Autodesk Inventor part; units mm, degrees
(part 2 of 2)
sketch "スケッチ3" plane through (0, 0, 5) normal (0, 0, 1) x (1, 0, 0)
  circle A0 centre (23.3432, 24.5782) radius 9 projected
  circle A1 centre (33.2427, 14.6787) radius 2.5 projected
  circle A2 centre (13.4437, 14.6787) radius 2.5 projected
  circle A3 centre (33.2427, 34.4777) radius 2.5 projected
  circle A4 centre (13.4437, 34.4777) radius 2.5 projected
  arc A5 (22.1602, 48.3922) -> (21.7942, 49.4809) centre (16.0401, 46.941) ccw projected
  arc A6 (21.7942, 49.4809) -> (20.6745, 51.446) centre (11.8398, 45.1102) ccw projected
  arc A7 (20.6745, 51.446) -> (19.2464, 51.2656) centre (23.3432, 24.5782) ccw projected
  arc A8 (19.2464, 51.2656) -> (18.6505, 49.0838) centre (29.3792, 47.3259) ccw projected
  arc A9 (18.6505, 49.0838) -> (18.5668, 47.9382) centre (24.8555, 48.0547) ccw projected
  arc A10 (18.5668, 47.9382) -> (18.5978, 47.5862) centre (20.8543, 47.962) ccw projected
  line L0 (18.5978, 47.5862) -> (18.7982, 46.6144) projected
  arc A11 (18.7982, 46.6144) -> (16.71, 46.0782) centre (23.3432, 24.5782) ccw projected
  line L1 (16.71, 46.0782) -> (16.4175, 47.0264) projected
  arc A12 (16.4175, 47.0264) -> (16.275, 47.3498) centre (14.259, 46.2687) ccw projected
  arc A13 (16.275, 47.3498) -> (15.6498, 48.3133) centre (10.7081, 44.4223) ccw projected
  arc A14 (15.6498, 48.3133) -> (14.0766, 49.9382) centre (7.0951, 41.6043) ccw projected
  arc A15 (14.0766, 49.9382) -> (12.7382, 49.4083) centre (23.3432, 24.5782) ccw projected
  arc A16 (12.7382, 49.4083) -> (12.7036, 47.1469) centre (23.5324, 48.1123) ccw projected
  arc A17 (12.7036, 47.1469) -> (12.9075, 46.0165) centre (18.9696, 47.6932) ccw projected
  arc A18 (12.9075, 46.0165) -> (13.025, 45.6833) centre (15.1172, 46.6084) ccw projected
  line L2 (13.025, 45.6833) -> (13.4608, 44.7918) projected
  arc A19 (13.4608, 44.7918) -> (11.5716, 43.7532) centre (23.3432, 24.5782) ccw projected
  line L3 (11.5716, 43.7532) -> (11.0524, 44.5988) projected
  arc A20 (11.0524, 44.5988) -> (10.834, 44.8766) centre (9.1502, 43.3281) ccw projected
  arc A21 (10.834, 44.8766) -> (9.9888, 45.6544) centre (6.1701, 40.6566) ccw projected
  arc A22 (9.9888, 45.6544) -> (8.0609, 46.837) centre (3.3713, 37.0287) ccw projected
  arc A23 (8.0609, 46.837) -> (6.8964, 45.9909) centre (23.3432, 24.5782) ccw projected
  arc A24 (6.8964, 45.9909) -> (7.4253, 43.7919) centre (17.6738, 47.42) ccw projected
  arc A25 (7.4253, 43.7919) -> (7.9038, 42.7477) centre (13.3585, 45.8793) ccw projected
  arc A26 (7.9038, 42.7477) -> (8.1005, 42.4542) centre (9.8969, 43.8706) ccw projected
  line L4 (8.1005, 42.4542) -> (8.7444, 41.6991) projected
  arc A27 (8.7444, 41.6991) -> (7.1728, 40.2233) centre (23.3432, 24.5782) ccw projected
  line L5 (7.1728, 40.2233) -> (6.4596, 40.9132) projected
  arc A28 (6.4596, 40.9132) -> (6.179, 41.128) centre (4.9332, 39.2093) ccw projected
  arc A29 (6.179, 41.128) -> (5.167, 41.6712) centre (2.7111, 35.8807) ccw projected
  arc A30 (5.167, 41.6712) -> (3.0055, 42.3371) centre (0.9025, 31.6707) ccw projected
  arc A31 (3.0055, 42.3371) -> (2.088, 41.228) centre (23.3432, 24.5782) ccw projected
  arc A32 (2.088, 41.228) -> (3.1471, 39.2296) centre (12.1714, 45.2925) ccw projected
  arc A33 (3.1471, 39.2296) -> (3.8703, 38.3373) centre (8.3748, 42.727) ccw projected
  arc A34 (3.8703, 38.3373) -> (4.1338, 38.1019) centre (5.5215, 39.9205) ccw projected
  line L6 (4.1338, 38.1019) -> (4.9452, 37.5306) projected
  arc A35 (4.9452, 37.5306) -> (3.7901, 35.7103) centre (23.3432, 24.5782) ccw projected
  line L7 (3.7901, 35.7103) -> (2.9277, 36.2013) projected
  arc A36 (2.9277, 36.2013) -> (2.6025, 36.3395) centre (1.873, 34.1713) ccw projected
  arc A37 (2.6025, 36.3395) -> (1.4872, 36.6139) centre (0.5485, 30.3946) ccw projected
  arc A38 (1.4872, 36.6139) -> (-0.772, 36.7214) centre (-0.1564, 25.8671) ccw projected
  arc A39 (-0.772, 36.7214) -> (-1.3849, 35.4189) centre (23.3432, 24.5782) ccw projected
  arc A40 (-1.3849, 35.4189) -> (0.138, 33.7468) centre (7.3709, 41.8634) ccw projected
  arc A41 (0.138, 33.7468) -> (1.0604, 33.0623) centre (4.3317, 38.4344) ccw projected
  arc A42 (1.0604, 33.0623) -> (1.3741, 32.8998) centre (2.266, 35.0064) ccw projected
  line L8 (1.3741, 32.8998) -> (2.3021, 32.5483) projected
  arc A43 (2.3021, 32.5483) -> (1.6359, 30.4979) centre (23.3432, 24.5782) ccw projected
  line L9 (1.6359, 30.4979) -> (0.6786, 30.759) projected
  arc A44 (0.6786, 30.759) -> (0.3292, 30.812) centre (0.1618, 28.5305) ccw projected
  arc A45 (0.3292, 30.812) -> (-0.8194, 30.8004) centre (-0.1819, 24.543) ccw projected
  arc A46 (-0.8194, 30.8004) -> (-3.0343, 30.3427) centre (0.2614, 19.9825) ccw projected
  arc A47 (-3.0343, 30.3427) -> (-3.304, 28.9287) centre (23.3432, 24.5782) ccw projected
  arc A48 (-3.304, 28.9287) -> (-1.4131, 27.6878) centre (3.5741, 37.3482) ccw projected
  arc A49 (-1.4131, 27.6878) -> (-0.3495, 27.2542) centre (1.4831, 33.2711) ccw projected
  arc A50 (-0.3495, 27.2542) -> (-0.0052, 27.1749) centre (0.3348, 29.4371) ccw projected
  line L10 (-0.0052, 27.1749) -> (0.9811, 27.0652) projected
  arc A51 (0.9811, 27.0652) -> (0.8457, 24.9135) centre (23.3432, 24.5782) ccw projected
  line L11 (0.8457, 24.9135) -> (-0.1465, 24.9283) projected
  arc A52 (-0.1465, 24.9283) -> (-0.4981, 24.8928) centre (-0.0928, 22.6413) ccw projected
  arc A53 (-0.4981, 24.8928) -> (-1.6076, 24.5959) centre (0.5659, 18.6937) ccw projected
  arc A54 (-1.6076, 24.5959) -> (-3.6391, 23.6018) centre (2.1295, 14.3867) ccw projected
  arc A55 (-3.6391, 23.6018) -> (-3.5487, 22.1652) centre (23.3432, 24.5782) ccw projected
  arc A56 (-3.5487, 22.1652) -> (-1.4087, 21.4335) centre (1.0194, 32.0306) ccw projected
  arc A57 (-1.4087, 21.4335) -> (-0.2706, 21.278) centre (0.008, 27.5616) ccw projected
  arc A58 (-0.2706, 21.278) -> (0.0826, 21.2868) centre (-0.1508, 23.5625) ccw projected
  line L12 (0.0826, 21.2868) -> (1.0651, 21.4258) projected
  arc A59 (1.0651, 21.4258) -> (1.4691, 19.3081) centre (23.3432, 24.5782) ccw projected
  line L13 (1.4691, 19.3081) -> (0.5044, 19.0757) projected
  arc A60 (0.5044, 19.0757) -> (0.1727, 18.9538) centre (1.1252, 16.8739) ccw projected
  arc A61 (0.1727, 18.9538) -> (-0.8282, 18.3903) centre (2.745, 13.2141) ccw projected
  arc A62 (-0.8282, 18.3903) -> (-2.5486, 16.9222) centre (5.3305, 9.4312) ccw projected
  arc A63 (-2.5486, 16.9222) -> (-2.1038, 15.5532) centre (23.3432, 24.5782) ccw projected
  arc A64 (-2.1038, 15.5532) -> (0.151, 15.3767) centre (-0.1326, 26.2447) ccw projected
  arc A65 (0.151, 15.3767) -> (1.292, 15.5092) centre (-0.0008, 21.6646) ccw projected
  arc A66 (1.292, 15.5092) -> (1.6319, 15.6055) centre (0.8399, 17.7517) ccw projected
  line L14 (1.6319, 15.6055) -> (2.549, 15.9845) projected
  arc A67 (2.549, 15.9845) -> (3.467, 14.0338) centre (23.3432, 24.5782) ccw projected
  line L15 (3.467, 14.0338) -> (2.5904, 13.5688) projected
  arc A68 (2.5904, 13.5688) -> (2.2994, 13.3682) centre (3.7392, 11.5905) ccw projected
  arc A69 (2.2994, 13.3682) -> (1.4701, 12.5736) centre (6.2182, 8.4485) ccw projected
  arc A70 (1.4701, 12.5736) -> (0.1688, 10.7237) centre (9.6633, 5.4275) ccw projected
  arc A71 (0.1688, 10.7237) -> (0.9401, 9.5083) centre (23.3432, 24.5782) ccw projected
  arc A72 (0.9401, 9.5083) -> (3.168, 9.8981) centre (0.1905, 20.3542) ccw projected
  arc A73 (3.168, 9.8981) -> (4.2401, 10.3102) centre (1.4572, 15.9507) ccw projected
  arc A74 (4.2401, 10.3102) -> (4.5454, 10.488) centre (3.2446, 12.3698) ccw projected
  line L16 (4.5454, 10.488) -> (5.3395, 11.0832) projected
  arc A75 (5.3395, 11.0832) -> (6.7137, 9.4221) centre (23.3432, 24.5782) ccw projected
  line L17 (6.7137, 9.4221) -> (5.9803, 8.7536) projected
  arc A76 (5.9803, 8.7536) -> (5.7483, 8.487) centre (7.585, 7.1232) ccw projected
  arc A77 (5.7483, 8.487) -> (5.1427, 7.5111) centre (10.7675, 4.6965) ccw projected
  arc A78 (5.1427, 7.5111) -> (4.3423, 5.3957) centre (14.8556, 2.6271) ccw projected
  arc A79 (4.3423, 5.3957) -> (5.3917, 4.4104) centre (23.3432, 24.5782) ccw projected
  arc A80 (5.3917, 4.4104) -> (7.4526, 5.342) centre (1.9683, 14.7291) ccw projected
  arc A81 (7.4526, 5.342) -> (8.3886, 6.0077) centre (4.2903, 10.7789) ccw projected
  arc A82 (8.3886, 6.0077) -> (8.6401, 6.2559) centre (6.9121, 7.7551) ccw projected
  line L18 (8.6401, 6.2559) -> (9.2611, 7.0298) projected
  arc A83 (9.2611, 7.0298) -> (11.0053, 5.7626) centre (23.3432, 24.5782) ccw projected
  line L19 (11.0053, 5.7626) -> (10.4612, 4.9328) projected
  arc A84 (10.4612, 4.9328) -> (10.3028, 4.6169) centre (12.4209, 3.7527) ccw projected
  arc A85 (10.3028, 4.6169) -> (9.9589, 3.521) centre (16.107, 2.1936) ccw projected
  arc A86 (9.9589, 3.521) -> (9.7098, 1.2731) centre (20.5813, 1.2059) ccw projected
  arc A87 (9.7098, 1.2731) -> (10.9712, 0.5796) centre (23.3432, 24.5782) ccw projected
  arc A88 (10.9712, 0.5796) -> (12.7357, 1.9945) centre (5.0893, 9.7228) ccw projected
  arc A89 (12.7357, 1.9945) -> (13.4767, 2.872) centre (8.3207, 6.4742) ccw projected
  arc A90 (13.4767, 2.872) -> (13.6586, 3.175) centre (11.6121, 4.1973) ccw projected
  line L20 (13.6586, 3.175) -> (14.0677, 4.0791) projected
  arc A91 (14.0677, 4.0791) -> (16.0722, 3.2854) centre (23.3432, 24.5782) ccw projected
  line L21 (16.0722, 3.2854) -> (15.7515, 2.3464) projected
  arc A92 (15.7515, 2.3464) -> (15.6767, 2.001) centre (17.9432, 1.6907) ccw projected
  arc A93 (15.6767, 2.001) -> (15.6161, 0.854) centre (21.9012, 1.0973) ccw projected
  arc A94 (15.6161, 0.854) -> (15.9339, -1.3853) centre (26.4805, 1.2534) ccw projected
  arc A95 (15.9339, -1.3853) -> (17.3281, -1.7432) centre (23.3432, 24.5782) ccw projected
  arc A96 (17.3281, -1.7432) -> (18.6853, 0.066) centre (9.3571, 5.6499) ccw projected
  arc A97 (18.6853, 0.066) -> (19.1848, 1.1003) centre (13.2949, 3.307) ccw projected
  arc A98 (19.1848, 1.1003) -> (19.2856, 1.439) centre (17.0492, 1.9202) ccw projected
  line L22 (19.2856, 1.439) -> (19.457, 2.4164) projected
  arc A99 (19.457, 2.4164) -> (21.5959, 2.1462) centre (23.3432, 24.5782) ccw projected
  line L23 (21.5959, 2.1462) -> (21.5188, 1.1568) projected
  arc A100 (21.5188, 1.1568) -> (21.5323, 0.8037) centre (23.8047, 1.0668) ccw projected
  arc A101 (21.5323, 0.8037) -> (21.7589, -0.3223) centre (27.7859, 1.4764) ccw projected
  arc A102 (21.7589, -0.3223) -> (22.6235, -2.4122) centre (32.1826, 2.7664) ccw projected
  arc A103 (22.6235, -2.4122) -> (24.0629, -2.4122) centre (23.3432, 24.5782) ccw projected
  arc A104 (24.0629, -2.4122) -> (24.9276, -0.3223) centre (14.5038, 2.7664) ccw projected
  arc A105 (24.9276, -0.3223) -> (25.1542, 0.8037) centre (18.9005, 1.4764) ccw projected
  arc A106 (25.1542, 0.8037) -> (25.1676, 1.1568) centre (22.8817, 1.0668) ccw projected
  line L24 (25.1676, 1.1568) -> (25.0905, 2.1462) projected
  arc A107 (25.0905, 2.1462) -> (27.2294, 2.4164) centre (23.3432, 24.5782) ccw projected
  line L25 (27.2294, 2.4164) -> (27.4008, 1.439) projected
  arc A108 (27.4008, 1.439) -> (27.5016, 1.1003) centre (29.6373, 1.9202) ccw projected
  arc A109 (27.5016, 1.1003) -> (28.0011, 0.066) centre (33.3915, 3.307) ccw projected
  arc A110 (28.0011, 0.066) -> (29.3583, -1.7432) centre (37.3293, 5.6499) ccw projected
  arc A111 (29.3583, -1.7432) -> (30.7526, -1.3853) centre (23.3432, 24.5782) ccw projected
  arc A112 (30.7526, -1.3853) -> (31.0703, 0.854) centre (20.2059, 1.2534) ccw projected
  arc A113 (31.0703, 0.854) -> (31.0098, 2.001) centre (24.7853, 1.0973) ccw projected
  arc A114 (31.0098, 2.001) -> (30.9349, 2.3464) centre (28.7433, 1.6907) ccw projected
  line L26 (30.9349, 2.3464) -> (30.6142, 3.2854) projected
  arc A115 (30.6142, 3.2854) -> (32.6188, 4.0791) centre (23.3432, 24.5782) ccw projected
  line L27 (32.6188, 4.0791) -> (33.0278, 3.175) projected
  arc A116 (33.0278, 3.175) -> (33.2097, 2.872) centre (35.0743, 4.1973) ccw projected
  arc A117 (33.2097, 2.872) -> (33.9507, 1.9945) centre (38.3658, 6.4742) ccw projected
  arc A118 (33.9507, 1.9945) -> (35.7152, 0.5796) centre (41.5972, 9.7228) ccw projected
  arc A119 (35.7152, 0.5796) -> (36.9766, 1.2731) centre (23.3432, 24.5782) ccw projected
  arc A120 (36.9766, 1.2731) -> (36.7275, 3.521) centre (26.1051, 1.2059) ccw projected
  arc A121 (36.7275, 3.521) -> (36.3836, 4.6169) centre (30.5794, 2.1936) ccw projected
  arc A122 (36.3836, 4.6169) -> (36.2252, 4.9328) centre (34.2655, 3.7527) ccw projected
  line L28 (36.2252, 4.9328) -> (35.6811, 5.7626) projected
  arc A123 (35.6811, 5.7626) -> (37.4253, 7.0298) centre (23.3432, 24.5782) ccw projected
  line L29 (37.4253, 7.0298) -> (38.0463, 6.2559) projected
  arc A124 (38.0463, 6.2559) -> (38.2978, 6.0077) centre (39.7743, 7.7551) ccw projected
  arc A125 (38.2978, 6.0077) -> (39.2338, 5.342) centre (42.3961, 10.7789) ccw projected
  arc A126 (39.2338, 5.342) -> (41.2948, 4.4104) centre (44.7181, 14.7291) ccw projected
  arc A127 (41.2948, 4.4104) -> (42.3441, 5.3957) centre (23.3432, 24.5782) ccw projected
  arc A128 (42.3441, 5.3957) -> (41.5437, 7.5111) centre (31.8308, 2.6271) ccw projected
  arc A129 (41.5437, 7.5111) -> (40.9381, 8.487) centre (35.9189, 4.6965) ccw projected
  arc A130 (40.9381, 8.487) -> (40.7062, 8.7536) centre (39.1015, 7.1232) ccw projected
  line L30 (40.7062, 8.7536) -> (39.9727, 9.4221) projected
  arc A131 (39.9727, 9.4221) -> (41.347, 11.0832) centre (23.3432, 24.5782) ccw projected
  line L31 (41.347, 11.0832) -> (42.141, 10.488) projected
  arc A132 (42.141, 10.488) -> (42.4463, 10.3102) centre (43.4418, 12.3698) ccw projected
  arc A133 (42.4463, 10.3102) -> (43.5185, 9.8981) centre (45.2292, 15.9507) ccw projected
  arc A134 (43.5185, 9.8981) -> (45.7463, 9.5083) centre (46.4959, 20.3542) ccw projected
  arc A135 (45.7463, 9.5083) -> (46.5176, 10.7237) centre (23.3432, 24.5782) ccw projected
  arc A136 (46.5176, 10.7237) -> (45.2163, 12.5736) centre (37.0232, 5.4275) ccw projected
  arc A137 (45.2163, 12.5736) -> (44.387, 13.3682) centre (40.4682, 8.4485) ccw projected
  arc A138 (44.387, 13.3682) -> (44.0961, 13.5688) centre (42.9473, 11.5905) ccw projected
  line L32 (44.0961, 13.5688) -> (43.2195, 14.0338) projected
  arc A139 (43.2195, 14.0338) -> (44.1374, 15.9845) centre (23.3432, 24.5782) ccw projected
  line L33 (44.1374, 15.9845) -> (45.0545, 15.6055) projected
  arc A140 (45.0545, 15.6055) -> (45.3945, 15.5092) centre (45.8465, 17.7517) ccw projected
  arc A141 (45.3945, 15.5092) -> (46.5354, 15.3767) centre (46.6872, 21.6646) ccw projected
  arc A142 (46.5354, 15.3767) -> (48.7902, 15.5532) centre (46.819, 26.2447) ccw projected
  arc A143 (48.7902, 15.5532) -> (49.235, 16.9222) centre (23.3432, 24.5782) ccw projected
  arc A144 (49.235, 16.9222) -> (47.5146, 18.3903) centre (41.356, 9.4312) ccw projected
  arc A145 (47.5146, 18.3903) -> (46.5137, 18.9538) centre (43.9415, 13.2141) ccw projected
  arc A146 (46.5137, 18.9538) -> (46.182, 19.0757) centre (45.5613, 16.8739) ccw projected
  line L34 (46.182, 19.0757) -> (45.2173, 19.3081) projected
  arc A147 (45.2173, 19.3081) -> (45.6213, 21.4258) centre (23.3432, 24.5782) ccw projected
  line L35 (45.6213, 21.4258) -> (46.6038, 21.2868) projected
  arc A148 (46.6038, 21.2868) -> (46.9571, 21.278) centre (46.8372, 23.5625) ccw projected
  arc A149 (46.9571, 21.278) -> (48.0951, 21.4335) centre (46.6784, 27.5616) ccw projected
  arc A150 (48.0951, 21.4335) -> (50.2352, 22.1652) centre (45.667, 32.0306) ccw projected
  arc A151 (50.2352, 22.1652) -> (50.3256, 23.6018) centre (23.3432, 24.5782) ccw projected
  arc A152 (50.3256, 23.6018) -> (48.2941, 24.5959) centre (44.557, 14.3867) ccw projected
  arc A153 (48.2941, 24.5959) -> (47.1845, 24.8928) centre (46.1205, 18.6937) ccw projected
  arc A154 (47.1845, 24.8928) -> (46.8329, 24.9283) centre (46.7792, 22.6413) ccw projected
  line L36 (46.8329, 24.9283) -> (45.8407, 24.9135) projected
  arc A155 (45.8407, 24.9135) -> (45.7053, 27.0652) centre (23.3432, 24.5782) ccw projected
  line L37 (45.7053, 27.0652) -> (46.6916, 27.1749) projected
  arc A156 (46.6916, 27.1749) -> (47.0359, 27.2542) centre (46.3517, 29.4371) ccw projected
  arc A157 (47.0359, 27.2542) -> (48.0995, 27.6878) centre (45.2034, 33.2711) ccw projected
  arc A158 (48.0995, 27.6878) -> (49.9904, 28.9287) centre (43.1124, 37.3482) ccw projected
  arc A159 (49.9904, 28.9287) -> (49.7207, 30.3427) centre (23.3432, 24.5782) ccw projected
  arc A160 (49.7207, 30.3427) -> (47.5058, 30.8004) centre (46.425, 19.9825) ccw projected
  arc A161 (47.5058, 30.8004) -> (46.3572, 30.812) centre (46.8683, 24.543) ccw projected
  arc A162 (46.3572, 30.812) -> (46.0079, 30.759) centre (46.5246, 28.5305) ccw projected
  line L38 (46.0079, 30.759) -> (45.0505, 30.4979) projected
  arc A163 (45.0505, 30.4979) -> (44.3843, 32.5483) centre (23.3432, 24.5782) ccw projected
  line L39 (44.3843, 32.5483) -> (45.3123, 32.8998) projected
  arc A164 (45.3123, 32.8998) -> (45.6261, 33.0623) centre (44.4205, 35.0064) ccw projected
  arc A165 (45.6261, 33.0623) -> (46.5484, 33.7468) centre (42.3548, 38.4344) ccw projected
  arc A166 (46.5484, 33.7468) -> (48.0713, 35.4189) centre (39.3155, 41.8634) ccw projected
  arc A167 (48.0713, 35.4189) -> (47.4584, 36.7214) centre (23.3432, 24.5782) ccw projected
  arc A168 (47.4584, 36.7214) -> (45.1993, 36.6139) centre (46.8428, 25.8671) ccw projected
  arc A169 (45.1993, 36.6139) -> (44.0839, 36.3395) centre (46.138, 30.3946) ccw projected
  arc A170 (44.0839, 36.3395) -> (43.7587, 36.2013) centre (44.8135, 34.1713) ccw projected
  line L40 (43.7587, 36.2013) -> (42.8964, 35.7103) projected
  arc A171 (42.8964, 35.7103) -> (41.7412, 37.5306) centre (23.3432, 24.5782) ccw projected
  line L41 (41.7412, 37.5306) -> (42.5526, 38.1019) projected
  arc A172 (42.5526, 38.1019) -> (42.8161, 38.3373) centre (41.1649, 39.9205) ccw projected
  arc A173 (42.8161, 38.3373) -> (43.5393, 39.2296) centre (38.3116, 42.727) ccw projected
  arc A174 (43.5393, 39.2296) -> (44.5985, 41.228) centre (34.5151, 45.2925) ccw projected
  arc A175 (44.5985, 41.228) -> (43.6809, 42.3371) centre (23.3432, 24.5782) ccw projected
  arc A176 (43.6809, 42.3371) -> (41.5195, 41.6712) centre (45.784, 31.6707) ccw projected
  arc A177 (41.5195, 41.6712) -> (40.5074, 41.128) centre (43.9754, 35.8807) ccw projected
  arc A178 (40.5074, 41.128) -> (40.2268, 40.9132) centre (41.7532, 39.2093) ccw projected
  line L42 (40.2268, 40.9132) -> (39.5136, 40.2233) projected
  arc A179 (39.5136, 40.2233) -> (37.942, 41.6991) centre (23.3432, 24.5782) ccw projected
  line L43 (37.942, 41.6991) -> (38.5859, 42.4542) projected
  arc A180 (38.5859, 42.4542) -> (38.7826, 42.7477) centre (36.7895, 43.8706) ccw projected
  arc A181 (38.7826, 42.7477) -> (39.2611, 43.7919) centre (33.3279, 45.8793) ccw projected
  arc A182 (39.2611, 43.7919) -> (39.7901, 45.9909) centre (29.0127, 47.42) ccw projected
  arc A183 (39.7901, 45.9909) -> (38.6255, 46.837) centre (23.3432, 24.5782) ccw projected
  arc A184 (38.6255, 46.837) -> (36.6976, 45.6544) centre (43.3151, 37.0287) ccw projected
  arc A185 (36.6976, 45.6544) -> (35.8524, 44.8766) centre (40.5163, 40.6566) ccw projected
  arc A186 (35.8524, 44.8766) -> (35.634, 44.5988) centre (37.5362, 43.3281) ccw projected
  line L44 (35.634, 44.5988) -> (35.1148, 43.7532) projected
  arc A187 (35.1148, 43.7532) -> (33.2256, 44.7918) centre (23.3432, 24.5782) ccw projected
  line L45 (33.2256, 44.7918) -> (33.6614, 45.6833) projected
  arc A188 (33.6614, 45.6833) -> (33.779, 46.0165) centre (31.5692, 46.6084) ccw projected
  arc A189 (33.779, 46.0165) -> (33.9828, 47.1469) centre (27.7168, 47.6932) ccw projected
  arc A190 (33.9828, 47.1469) -> (33.9482, 49.4083) centre (23.154, 48.1123) ccw projected
  arc A191 (33.9482, 49.4083) -> (32.6099, 49.9382) centre (23.3432, 24.5782) ccw projected
  arc A192 (32.6099, 49.9382) -> (31.0366, 48.3133) centre (39.5914, 41.6043) ccw projected
  arc A193 (31.0366, 48.3133) -> (30.4114, 47.3498) centre (35.9783, 44.4223) ccw projected
  arc A194 (30.4114, 47.3498) -> (30.2689, 47.0264) centre (32.4274, 46.2687) ccw projected
  line L46 (30.2689, 47.0264) -> (29.9764, 46.0782) projected
  arc A195 (29.9764, 46.0782) -> (27.8882, 46.6144) centre (23.3432, 24.5782) ccw projected
  line L47 (27.8882, 46.6144) -> (28.0887, 47.5862) projected
  arc A196 (28.0887, 47.5862) -> (28.1196, 47.9382) centre (25.8321, 47.962) ccw projected
  arc A197 (28.1196, 47.9382) -> (28.0359, 49.0838) centre (21.831, 48.0547) ccw projected
  arc A198 (28.0359, 49.0838) -> (27.4401, 51.2656) centre (17.3073, 47.3259) ccw projected
  arc A199 (27.4401, 51.2656) -> (26.012, 51.446) centre (23.3432, 24.5782) ccw projected
  arc A200 (26.012, 51.446) -> (24.8922, 49.4809) centre (34.8467, 45.1102) ccw projected
  arc A201 (24.8922, 49.4809) -> (24.5263, 48.3922) centre (30.6463, 46.941) ccw projected
  arc A202 (24.5263, 48.3922) -> (24.4687, 48.0435) centre (26.7478, 47.8464) ccw projected
  line L48 (24.4687, 48.0435) -> (24.4212, 47.0524) projected
  arc A203 (24.4212, 47.0524) -> (22.2653, 47.0524) centre (23.3432, 24.5782) ccw projected
  line L49 (22.2653, 47.0524) -> (22.2177, 48.0435) projected
  arc A204 (22.2177, 48.0435) -> (22.1602, 48.3922) centre (19.9386, 47.8464) ccw projected
  circle A205 centre (23.3432, 24.5782) radius 19.4
  circle A206 centre (23.3432, 24.5782) radius 12
  circle A207 centre (13.4437, 34.4777) radius 5.5
  circle A208 centre (33.2427, 34.4777) radius 5.5
  circle A209 centre (33.2427, 14.6787) radius 5.5
  circle A210 centre (13.4437, 14.6787) radius 5.5
  point P0 (0, 0)
  point P1 (37.9022, 11.7565)
  point P2 (37.9022, 37.4)
  point P3 (34.4535, 29.1126)
  point P4 (34.4535, 20.0438)
  point P5 (18.8088, 13.4679)
  point P6 (10.5215, 10.0193)
  point P7 (36.165, 10.0193)
  point P8 (27.8776, 13.4679)
  point P9 (8.7843, 11.7565)
  point P10 (12.2329, 20.0438)
  point P11 (12.2329, 29.1126)
  point P12 (8.7843, 37.4)
  point P13 (27.8776, 35.6885)
  point P14 (36.165, 39.1371)
  point P15 (10.5215, 39.1371)
  point P16 (18.8088, 35.6885)
  dimension "d10" = 3.1
  dimension "d11" = 3
  dimension "d12" = 3
  dimension "d13" = 3
  dimension "d14" = 3
  dimension "d15" = 3
  constraints: 6 centre point, 1 coincident
  measures "d10" radial gap between concentric circles of A203 A205
  measures "d11" radial gap between concentric circles of A0 A206
  measures "d12" radial gap between concentric circles of A4 A207
  measures "d13" radial gap between concentric circles of A3 A208
  measures "d14" radial gap between concentric circles of A1 A209
  measures "d15" radial gap between concentric circles of A2 A210
extrude "押し出し3" cut sketch "スケッチ3" against normal blind 5 contours A208 A205 A209 A206 | A206 A207 A205 A208 | A209 A205 A210 A206 | A206 A210 A205 A207
fillet "フィレット1" radius 2 16 edges at (8.7843, 37.4, 2.5) (10.5215, 39.1371, 2.5) (36.165, 39.1371, 2.5) (37.9022, 37.4, 2.5) (36.165, 10.0193, 2.5) (37.9022, 11.7565, 2.5) (10.5215, 10.0193, 2.5) (8.7843, 11.7565, 2.5) (18.8088, 13.4679, 2.5) (12.2329, 20.0438, 2.5) (12.2329, 29.1126, 2.5) (18.8088, 35.6885, 2.5) (27.8776, 35.6885, 2.5) (34.4535, 29.1126, 2.5) (27.8776, 13.4679, 2.5) (34.4535, 20.0438, 2.5)
